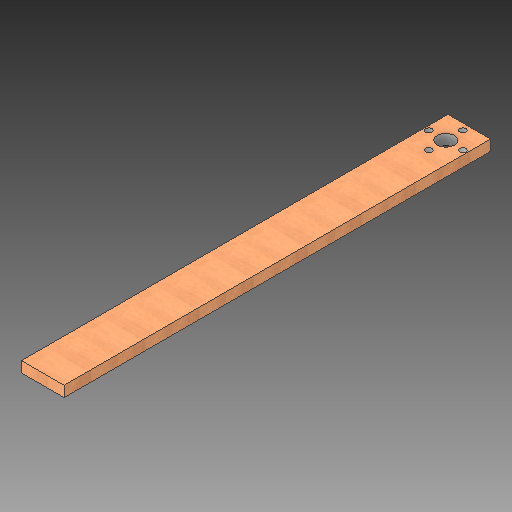
# Autodesk Inventor part: bras-lanceur
Saved by Autodesk Inventor 2019 (Build 230136000, 136)
## iProperties
Created: 2018-04-02
Part Number: bras-lanceur
Material: Générique
Document SubType Name: Modeling
Designer: franc
Density: 1 g/cm^3
Appearance: Par défaut
Author: franc
Autodesk Inventor part; units mm, degrees
ref_plane "YZ Plane" through (0, 0, 0) normal (1, 0, 0) x (0, 1, 0)
ref_plane "XZ Plane" through (0, 0, 0) normal (0, 1, 0) x (-1, 0, 0)
ref_plane "XY Plane" through (0, 0, 0) normal (0, 0, 1) x (1, 0, 0)
sketch "Esquisse1" plane through (0, 0, 0) normal (0, 1, 0) x (-1, 0, 0)
  line L0 (23.7435, 85.6153) -> (3.7435, 85.6153)
  line L1 (3.7435, 85.6153) -> (3.7435, -114.3847)
  line L2 (3.7435, -114.3847) -> (23.7435, -114.3847)
  line L3 (23.7435, -114.3847) -> (23.7435, 85.6153)
  point P0 (0, 0)
  dimension "d0" = 200
  dimension "d1" = 20
  constraints: 8 end point, 2 parallel, 1 horizontal, 1 perpendicular
  measures "d0" distance of L2.end L0.start
  measures "d1" distance of L0.start L0.end
extrude "Extrusion1" add sketch "Esquisse1" along normal blind 5
sketch "Esquisse2" plane through (0, 5, 0) normal (0, 1, 0) x (1, 0, 0)
  circle A0 centre (-13.7435, 103.3847) radius 4
  line L0 (-3.7435, 114.3847) -> (-23.7435, 114.3847) projected
  line L1 (-3.7435, -85.6153) -> (-3.7435, 114.3847) projected
  circle A1 centre (-13.7435, 111.3847) radius 1.5
  circle A2 centre (-5.7435, 103.3847) radius 1.5
  circle A3 centre (-21.7435, 103.3847) radius 1.5
  line L2 (-23.7435, 114.3847) -> (-23.7435, -85.6153) projected
  circle A4 centre (-13.7435, 95.3847) radius 1.5
  point P0 (0, 0)
  dimension "d4" = 11
  dimension "d5" = 10
  dimension "d6" = 8
  dimension "d9" = 3
  dimension "d10" = 3
  dimension "d11" = 10
  dimension "d12" = 2
  dimension "d13" = 3
  dimension "d14" = 11
  dimension "d15" = 2
  dimension "d16" = 11
  dimension "d17" = 3
  dimension "d18" = 10
  dimension "d19" = 3
  dimension "d20" = 19
  constraints: 5 centre point
  measures "d4" distance from line of L0 A0.centre
  measures "d5" distance from line of L1 A0.centre
  measures "d6" diameter of A0
  measures "d9" diameter of A1
  measures "d10" distance from line of L0 A1.centre
  measures "d11" distance from line of L1 A1.centre
  measures "d12" distance from line of L1 A2.centre
  measures "d13" diameter of A2
  measures "d14" distance from line of L0 A2.centre
  measures "d15" distance from line of L2 A3.centre
  measures "d16" distance from line of L0 A3.centre
  measures "d17" diameter of A3
  measures "d18" distance from line of L1 A4.centre
  measures "d19" diameter of A4
  measures "d20" distance from line of L0 A4.centre
extrude "Extrusion2" cut sketch "Esquisse2" against normal through all
